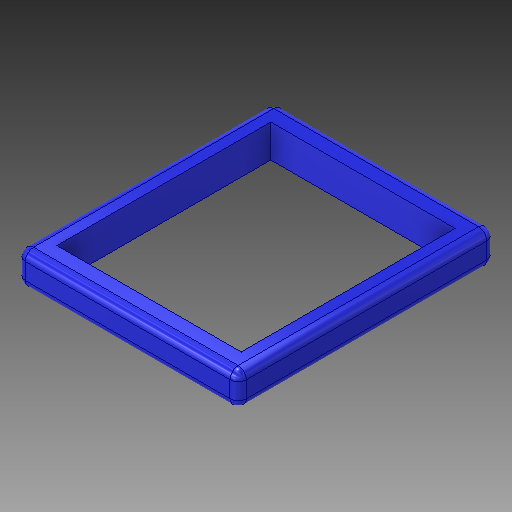
# Autodesk Inventor part: bumpers
Saved by Autodesk Inventor 2017 SP1 (Build 210196100, 196)
## iProperties
Created: 2018-01-18
Part Number: bumpers
Material: Generic
Document SubType Name: Modeling
Designer: Ben
Density: 1 g/cm^3
Appearance: Blue - Wall Paint - Glossy
Mass: 31144.2 g
Surface Area: 12667.7 cm^2
Volume: 31144.2 cm^3
Author: Ben
Autodesk Inventor part; units mm, degrees
ref_plane "YZ Plane" through (0, 0, 0) normal (1, 0, 0) x (0, 1, 0)
ref_plane "XZ Plane" through (0, 0, 0) normal (0, 1, 0) x (-1, 0, 0)
ref_plane "XY Plane" through (0, 0, 0) normal (0, 0, 1) x (1, 0, 0)
sketch "Sketch1" plane through (0, 0, 0) normal (0, 1, 0) x (-1, 0, 0)
  line L0 (-355.6, 412.75) -> (355.6, 412.75)
  line L1 (355.6, 412.75) -> (355.6, -412.75)
  line L2 (355.6, -412.75) -> (-355.6, -412.75)
  line L3 (-355.6, -412.75) -> (-355.6, 412.75)
  line L4 (-355.6, 412.75) -> (355.6, -412.75) construction
  line L5 (355.6, 412.75) -> (-355.6, -412.75) construction
  line L6 (-426.72, 495.3) -> (426.72, 495.3)
  line L7 (426.72, 495.3) -> (426.72, -495.3)
  line L8 (426.72, -495.3) -> (-426.72, -495.3)
  line L9 (-426.72, -495.3) -> (-426.72, 495.3)
  line L10 (-426.72, 495.3) -> (426.72, -495.3) construction
  line L11 (426.72, 495.3) -> (-426.72, -495.3) construction
  point P0 (0, 0)
  dimension "d0" = 825.5
  dimension "d1" = 711.2
  dimension "d2" = 82.55
  constraints: 24 end point, 4 midpoint, 4 parallel, 2 horizontal, 2 perpendicular, 1 point on line
  measures "d0" distance of L0.end L1.end
  measures "d1" distance of L1.end L2.end
  measures "d2" distance between parallel lines of L2 L8
extrude "Extrusion1" add sketch "Sketch1" along normal blind 127
fillet "Fillet1" radius 31.75 12 edges at (426.72, 127, 0) (0, 127, 495.3) (-426.72, 127, 0) (0, 127, -495.3) (426.72, 0, 0) (0, 0, 495.3) (0, 0, -495.3) (426.72, 63.5, -495.3) (426.72, 63.5, 495.3) (-426.72, 63.5, -495.3) (-426.72, 0, 0) (-426.72, 63.5, 495.3)
body "Solid1"
